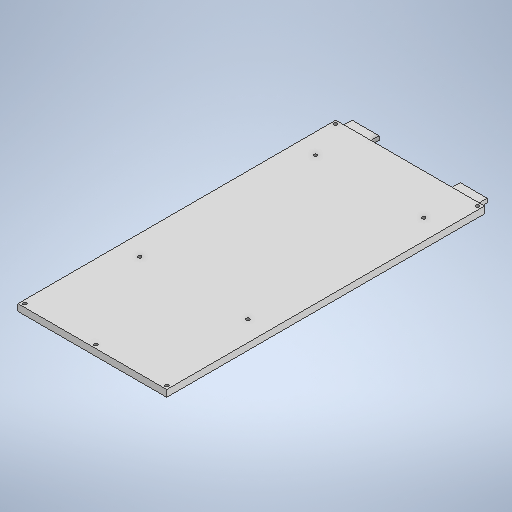
# Autodesk Inventor part: chassis_bas
Saved by Autodesk Inventor 2026.2 (Build 302298010, 298A)
## iProperties
Created: 2026-03-16
Part Number: chassis_bas
Material: Générique
Document SubType Name: Modeling
Designer: genon
Density: 1 g/cm^3
Appearance: Par défaut
Author: genon
Autodesk Inventor part; units mm, degrees
ref_plane "YZ Plane" through (0, 0, 0) normal (1, 0, 0) x (0, 1, 0)
ref_plane "XZ Plane" through (0, 0, 0) normal (0, 1, 0) x (-1, 0, 0)
ref_plane "XY Plane" through (0, 0, 0) normal (0, 0, 1) x (1, 0, 0)
sketch "Esquisse1" plane through (0, 0, 0) normal (0, 1, 0) x (-1, 0, 0)
  line L0 (55, -100) -> (-55, -100)
  line L1 (-55, -100) -> (-55, 100)
  line L2 (-55, 100) -> (55, 100)
  line L3 (55, 100) -> (55, -100)
  line L4 (55, -100) -> (-55, 100) construction
  line L5 (-55, -100) -> (55, 100) construction
  point P0 (0, 0)
  dimension "d0" = 110
  dimension "d1" = 200
  constraints: 12 end point, 2 midpoint, 2 parallel, 1 horizontal, 1 perpendicular
  measures "d0" distance of L1.end L2.end
  measures "d1" distance of L0.end L1.end
extrude "Extrusion1" add sketch "Esquisse1" along normal blind 5
sketch "Esquisse6" plane through (-55, 0, 100) normal (0, 0, 1) x (1, 0, 0)
  line L0 (0, 0) -> (110, 0) projected
  line L1 (110, 0) -> (110, 5) projected
  line L2 (0, 5) -> (110, 5) projected
  line L3 (0, 0) -> (0, 5) projected
  point P0 (55, 0)
extrude "Extrusion2" add sketch "Esquisse6" along normal blind 40
sketch "Esquisse3" plane through (0, 0, 0) normal (0, -1, 0) x (1, 0, 0)
  line L0 (0, 0) -> (52.5, 0)
  line L1 (52.5, 0) -> (52.5, -97.5)
  line L2 (0, 28.6272) -> (0, -29.3855)
  line L3 (0, 0) -> (0, 137.5)
  line L4 (0, 137.5) -> (52.5, 137.5)
  point P0 (-52.5, -97.5)
  point P1 (-52.5, 137.5)
  dimension "d18" = 52.5
  dimension "d19" = 97.5
  dimension "d49" = 137.5
  dimension "d50" = 52.5
  constraints: 10 end point, 2 coincident, 2 perpendicular, 2 symmetric about line, 2 vertical, 1 horizontal
  measures "d18" distance of L0.start L0.end
  measures "d19" distance of L0.end L1.end
  measures "d49" distance of L0.start L3.end
  measures "d50" distance of L3.end L4.end
hole "Perçage2" at (52.5, 0, -97.5) at (-52.5, 0, -97.5) at (-52.5, 0, 137.5) at (52.5, 0, 137.5) direction (0, 1, 0) diameter 2.459 end through all thread size "M3x0.5" class "6H" standard "ISO Metric profile"
sketch "Esquisse5" plane through (0, 5, 0) normal (0, 1, 0) x (1, 0, 0)
  line L0 (0, 0) -> (-40, 0)
  line L1 (-40, 0) -> (-40, 65)
  line L2 (-40, 65) -> (40, 65)
  line L3 (40, 65) -> (40, -65)
  line L4 (40, -65) -> (-40, -65)
  line L5 (-40, -65) -> (-40, 0)
  dimension "d36" = 40
  dimension "d37" = 65
  dimension "d38" = 80
  dimension "d39" = 130
  constraints: 12 end point, 5 perpendicular, 4 coincident, 1 horizontal, 1 point on line
  measures "d36" distance of L0.start L0.end
  measures "d37" distance of L0.end L1.end
  measures "d38" distance of L1.end L2.end
  measures "d39" distance of L2.end L3.end
hole "Perçage4" at (-40, 5, -65) at (40, 5, -65) at (40, 5, 65) at (-40, 5, 65) direction (0, -1, 0) diameter 2.459 end through all thread size "M3x0.5" class "6H" standard "ISO Metric profile"
sketch "Esquisse4" plane through (0, 0, 0) normal (0, -1, 0) x (1, 0, 0)
  line L0 (0, 0) -> (0, 137.5)
  line L1 (0, 0) -> (87.5, 0)
  line L2 (0, 0) -> (0, -97.5)
  line L3 (55, -100) -> (-55, -100) projected
  point P0 (-87.5, 0)
  dimension "d27" = 137.5
  dimension "d28" = 87.5
  dimension "d51" = 97.5
  constraints: 6 end point, 3 coincident, 1 horizontal, 1 perpendicular, 1 symmetric about line, 1 vertical
  measures "d27" distance of L0.start L0.end
  measures "d28" distance of L0.start L1.end
  measures "d51" distance of L0.start L2.end
hole "Perçage3" at (87.5, 0, 0) at (0, 0, 137.5) at (-87.5, 0, 0) at (0, 0, -97.5) direction (0, 1, 0) diameter 2.459 end through all thread size "M3x0.5" class "6H" standard "ISO Metric profile"
sketch "Esquisse7" plane through (0, 5, 0) normal (0, 1, 0) x (1, 0, 0)
  line L0 (55, 100) -> (-55, 100) projected
  line L1 (55, 100) -> (55, -140) projected
  line L2 (-55, 100) -> (55, 100)
  line L3 (55, 100) -> (55, 95)
  line L4 (55, 95) -> (-55, 95)
  line L5 (-55, 95) -> (-55, 100)
  point P0 (0, 0)
  dimension "d52" = 5
  constraints: 8 end point, 2 parallel, 1 horizontal, 1 perpendicular, 1 point on line
  measures "d52" distance of L2.end L3.end
extrude "Extrusion3" cut sketch "Esquisse7" against normal blind 10
sketch "Esquisse8" plane through (0, 5, 0) normal (0, 1, 0) x (1, 0, 0)
  line L0 (-55, 95) -> (-55, -140) projected
  line L1 (-55, 95) -> (-55, 92.5)
  line L2 (-55, 92.5) -> (-52.5, 92.5)
  line L3 (55, 95) -> (55, -140) projected
  line L4 (55, 95) -> (52.5, 95)
  line L5 (-55, 95) -> (55, 95) projected
  line L6 (52.5, 95) -> (52.5, 92.5)
  point P0 (0, 0)
  dimension "d55" = 2.5
  dimension "d56" = 2.5
  dimension "d57" = 2.5
  constraints: 8 end point, 2 coincident, 2 perpendicular, 2 point on line
  measures "d55" distance of L0.start L1.end
  measures "d56" distance of L1.end L2.end
  measures "d57" distance of L3.start L4.end
hole "Perçage5" at (-52.5, 5, -92.5) at (52.5, 5, -92.5) direction (0, -1, 0) diameter 2.459 end through all thread size "M3x0.5" class "6H" standard "ISO Metric profile"
sketch "Esquisse9" plane through (55, 5, -95) normal (0, 0, -1) x (-1, 0, 0)
  line L0 (0, -5) -> (0, 0) projected
  line L1 (0, 0) -> (5, 0)
  line L2 (0, 0) -> (110, 0) projected
  line L3 (5, 0) -> (5, -1)
  line L4 (5, -1) -> (25, -1)
  line L5 (25, -1) -> (25, -4)
  line L6 (25, -4) -> (5, -4)
  line L7 (5, -4) -> (5, -1)
  line L8 (110, 0) -> (105, 0)
  line L9 (105, 0) -> (105, -1)
  line L10 (105, -1) -> (85, -1)
  line L11 (85, -1) -> (85, -4)
  line L12 (85, -4) -> (105, -4)
  line L13 (105, -4) -> (105, -1)
  point P0 (55, -5)
  dimension "d65" = 5
  dimension "d66" = 1
  dimension "d67" = 20
  dimension "d68" = 3
  dimension "d69" = 5
  dimension "d70" = 20
  constraints: 24 end point, 4 parallel, 4 perpendicular, 2 horizontal, 2 point on line
  measures "d65" distance of L0.end L1.end
  measures "d66" distance of L1.end L3.end
  measures "d67" distance of L5.end L6.end
  measures "d68" distance of L4.end L5.end
  measures "d69" distance of L2.end L8.end
  measures "d70" distance of L12.end L11.end
extrude "Extrusion4" add sketch "Esquisse9" along normal blind 7
